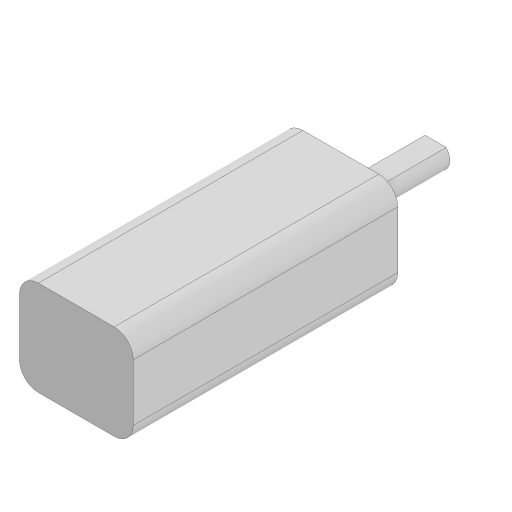
# Autodesk Inventor part: motor
Saved by Autodesk Inventor 2023 (Build 270158000, 158)
## iProperties
Created: 2023-04-25
Part Number: motor
Material: Generic
Document SubType Name: Modeling
Designer: Juyoung Han
Density: 1 g/cm^3
Appearance: Default
Author: Juyoung Han
Autodesk Inventor part; units mm, degrees
ref_plane "YZ Plane" through (0, 0, 0) normal (1, 0, 0) x (0, 1, 0)
ref_plane "XZ Plane" through (0, 0, 0) normal (0, 1, 0) x (-1, 0, 0)
ref_plane "XY Plane" through (0, 0, 0) normal (0, 0, 1) x (1, 0, 0)
sketch "Sketch1" plane through (0, 0, 0) normal (0, 0, 1) x (1, 0, 0)
  line L0 (0, 0) -> (-12, 0)
  line L1 (-12, 0) -> (-12, 10)
  line L2 (-12, 10) -> (0, 10)
  line L3 (0, 10) -> (0, 0)
  dimension "d0" = 12
  dimension "d1" = 10
  constraints: 8 end point, 2 parallel, 1 horizontal, 1 perpendicular
  measures "d0" distance of L1.end L2.end
  measures "d1" distance of L0.end L1.end
extrude "Extrusion1" add sketch "Sketch1" along normal blind 27.9
sketch "Sketch2" plane through (0, 0, 0) normal (0, 0, -1) x (-1, 0, 0)
  circle A0 centre (6, 5) radius 2
  line L0 (12, 0) -> (0, 0) projected
  line L1 (0, 0) -> (0, 10) projected
  point P0 (6, 0)
  dimension "d4" = 5
  dimension "d5" = 6
  dimension "d9" = 4
  constraints: 1 centre point, 1 midpoint
  measures "d4" distance of A0.centre point (6, 0)
  measures "d5" distance from line of L1 A0.centre
  measures "d9" diameter of A0
extrude "Extrusion2" add sketch "Sketch2" along normal blind 0.7
sketch "Sketch5" plane through (-6, 5, -0.7) normal (0, 0, -1) x (-1, 0, 0)
  circle A0 centre (0, 0) radius 2 projected
  arc A1 (-1.118, 1) -> (1.118, 1) centre (0, 0) ccw
  line L0 (-1.118, 1) -> (1.118, 1)
  point P0 (-6, -5)
  point P1 (0.4397, 1)
  dimension "d14" = 3
  dimension "d15" = 1
  constraints: 2 end point, 2 point on circle, 1 centre point, 1 coincident, 1 horizontal, 1 point on line
  measures "d14" diameter of A1
  measures "d15" vertical distance of A0.centre point (0.44, 1)
extrude "Extrusion4" add sketch "Sketch5" along normal blind 9.3 contours L0 A1
fillet "Fillet1" radius 2 4 edges at (-12, 10, 13.95) (0, 10, 13.95) (-12, 0, 13.95) (0, 0, 13.95)
body "Solid1"
